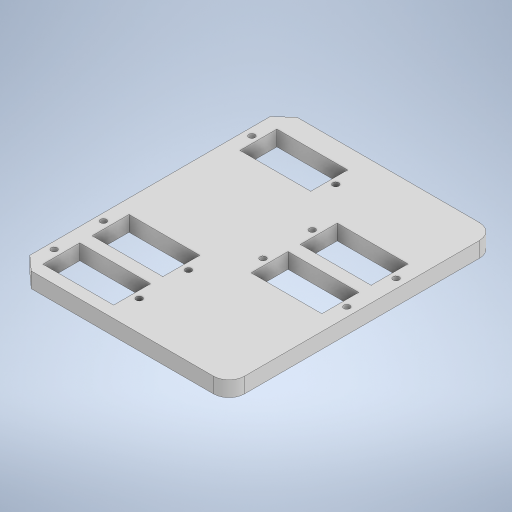
# Autodesk Inventor part: Robotic Hand Tray
Saved by Autodesk Inventor 2023 (Build 270158000, 158)
## iProperties
Created: 2023-03-10
Part Number: Robotic Hand Tray
Material: Generic
Document SubType Name: Modeling
Designer: 1senadi
Density: 1 g/cm^3
Appearance: Default
Author: 1senadi
Autodesk Inventor part; units mm, degrees
ref_plane "YZ Plane" through (0, 0, 0) normal (1, 0, 0) x (0, 1, 0)
ref_plane "XZ Plane" through (0, 0, 0) normal (0, 1, 0) x (-1, 0, 0)
ref_plane "Work Plane2" through (0, 5.93, 0) normal (0, 1, 0) x (1, 0, 0)
sketch "Sketch7" plane through (0, 5.93, 0) normal (0, 1, 0) x (1, 0, 0)
  line L0 (-68.89, 72.25) -> (-68.89, 75.38) projected
  line L1 (-70.59, 75.38) -> (-68.89, 75.38) projected
  line L2 (-70.59, 83.0068) -> (-70.59, 75.38) projected
  line L3 (-64.9127, 88.12) -> (-70.59, 83.0068) projected
  line L4 (-5, 88.12) -> (-64.9127, 88.12) projected
  arc A0 (1.7, 81.42) -> (-5, 88.12) centre (-5, 81.42) ccw projected
  line L5 (1.7, 5) -> (1.7, 81.42) projected
  arc A1 (-5, -1.7) -> (1.7, 5) centre (-5, 5) ccw projected
  line L6 (-64.9127, -1.7) -> (-5, -1.7) projected
  line L7 (-70.59, 3.4132) -> (-64.9127, -1.7) projected
  line L8 (-70.59, 14.5) -> (-70.59, 3.4132) projected
  line L9 (-68.89, 14.5) -> (-70.59, 14.5) projected
  line L10 (-68.89, 14.5) -> (-68.89, 17.63) projected
  line L11 (-70.59, 17.63) -> (-68.89, 17.63) projected
  line L12 (-70.59, 47.6) -> (-70.59, 17.63) projected
  line L13 (-68.89, 47.6) -> (-70.59, 47.6) projected
  line L14 (-68.89, 47.6) -> (-68.89, 50.73) projected
  line L15 (-70.59, 50.73) -> (-68.89, 50.73) projected
  line L16 (-70.59, 72.25) -> (-70.59, 50.73) projected
  line L17 (-68.89, 72.25) -> (-70.59, 72.25) projected
  line L18 (5.3534, 92.34) -> (10.14, 87.0271) projected
  line L19 (-69.6869, 92.34) -> (5.3534, 92.34) projected
  line L20 (-73.78, 86.0365) -> (-69.6869, 92.34) projected
  line L21 (-73.78, 75.38) -> (-73.78, 86.0365) projected
  line L22 (-73.78, 75.38) -> (-73.78, 72.25) projected
  line L23 (-73.78, 50.73) -> (-73.78, 72.25) projected
  line L24 (-73.78, 50.73) -> (-73.78, 47.6) projected
  line L25 (-73.78, 17.63) -> (-73.78, 47.6) projected
  line L26 (-73.78, 17.63) -> (-73.78, 14.5) projected
  line L27 (-73.78, -2.6865) -> (-73.78, 14.5) projected
  line L28 (-69.6869, -8.99) -> (-73.78, -2.6865) projected
  line L29 (4.8271, -8.99) -> (-69.6869, -8.99) projected
  line L30 (10.14, -4.2034) -> (4.8271, -8.99) projected
  line L31 (10.14, 87.0271) -> (10.14, -4.2034) projected
  line L32 (-5, 0) -> (-64.26, 0) projected
  line L33 (-68.89, 4.17) -> (-64.26, 0) projected
  line L34 (-68.89, 4.17) -> (-68.89, 14.5) projected
  line L35 (-68.89, 17.63) -> (-68.89, 47.6) projected
  line L36 (-68.89, 50.73) -> (-68.89, 72.25) projected
  line L37 (-68.89, 75.38) -> (-68.89, 82.25) projected
  line L38 (-64.26, 86.42) -> (-68.89, 82.25) projected
  line L39 (-64.26, 86.42) -> (-5, 86.42) projected
  arc A2 (0, 81.42) -> (-5, 86.42) centre (-5, 81.42) ccw projected
  line L40 (0, 81.42) -> (0, 5) projected
  arc A3 (-5, 0) -> (0, 5) centre (-5, 5) ccw projected
  line L41 (-68.89, 14.5) -> (-70.59, 14.5) projected
  line L42 (-68.89, 14.5) -> (-68.89, 75.38)
  point P0 (0, 0)
  constraints: 2 end point, 1 collinear
extrude "Extrusion6" add sketch "Sketch7" along normal blind 5 contours L0 L37 L38 L39 A2 L40 A3 L32 L33 L34 L10 L35 L14 L36
sketch "Sketch8" plane through (0, 10.93, 0) normal (0, 1, 0) x (1, 0, 0)
  line L0 (-64.26, 0) -> (-64.26, 16.2)
  line L1 (-64.26, 16.2) -> (-64.26, 17.765)
  line L2 (-64.26, 17.765) -> (-41.26, 17.765)
  line L3 (-64.26, 17.765) -> (-64.26, 15.765)
  line L4 (-64.26, 15.765) -> (-41.26, 15.765)
  line L5 (-41.26, 15.765) -> (-41.26, 3.765)
  line L6 (-41.26, 3.765) -> (-64.26, 3.765)
  line L7 (-64.26, 3.765) -> (-64.26, 15.765)
  line L8 (-64.26, 9.765) -> (-66.573, 9.765)
  circle A0 centre (-66.573, 9.765) radius 1
  line L9 (-41.26, 9.765) -> (-38.947, 9.765)
  circle A1 centre (-38.947, 9.765) radius 1
  line L10 (-64.26, 17.765) -> (-64.26, 19.765)
  line L11 (-64.26, 19.765) -> (-41.26, 19.765)
  line L12 (-41.26, 19.765) -> (-41.26, 31.765)
  line L13 (-41.26, 31.765) -> (-64.26, 31.765)
  line L14 (-64.26, 31.765) -> (-64.26, 19.765)
  line L15 (-64.26, 25.765) -> (-66.573, 25.765)
  circle A2 centre (-66.573, 25.765) radius 1
  line L16 (-41.26, 25.765) -> (-38.947, 25.765)
  circle A3 centre (-38.947, 25.765) radius 1
  point P0 (0, 0)
  dimension "d56" = 16.2
  dimension "d57" = 1.565
  dimension "d58" = 23
  dimension "d59" = 90
  dimension "d60" = 2
  dimension "d61" = 23
  dimension "d62" = 12
  dimension "d63" = 2.313
  dimension "d64" = 2
  dimension "d65" = 2.313
  dimension "d66" = 2
  dimension "d67" = 2
  dimension "d68" = 23
  dimension "d69" = 12
  dimension "d70" = 2.313
  dimension "d71" = 2
  dimension "d73" = 2
  constraints: 34 end point, 6 horizontal, 4 centre point, 4 coincident, 4 midpoint, 4 parallel, 3 perpendicular, 3 vertical, 1 point on line
  measures "d56" distance of L0.start L0.end
  measures "d57" distance of L0.end L1.end
  measures "d58" distance of L1.end L2.end
  measures "d59" angle of L1 L2
  measures "d60" distance of L1.end L3.end
  measures "d61" distance of L5.end L6.end
  measures "d62" distance of L4.end L5.end
  measures "d63" distance of L8.start L8.end
  measures "d64" diameter of A0
  measures "d65" distance of L9.start L9.end
  measures "d66" diameter of A1
  measures "d67" distance of L1.end L10.end
  measures "d68" distance of L13.end L12.end
  measures "d69" distance of L12.end L11.end
  measures "d70" distance of L15.start L15.end
  measures "d71" diameter of A2
  measures "d73" diameter of A3
extrude "Extrusion7" cut sketch "Sketch8" against normal up to surface (5 mm away)
sketch "Sketch9" plane through (0, 10.93, 0) normal (0, 1, 0) x (1, 0, 0)
  line L0 (-5, 86.42) -> (-64.26, 86.42) projected
  line L1 (-64.26, 86.42) -> (-64.26, 75.38)
  line L2 (-64.26, 75.38) -> (-64.26, 73.815)
  line L3 (-64.26, 73.815) -> (-64.26, 79.815)
  line L4 (-64.26, 79.815) -> (-41.26, 79.815)
  line L5 (-64.26, 73.815) -> (-66.39, 73.815)
  circle A0 centre (-66.39, 73.815) radius 1
  line L6 (-41.26, 79.815) -> (-41.26, 67.815)
  line L7 (-41.26, 67.815) -> (-64.26, 67.815)
  line L8 (-64.26, 67.815) -> (-64.26, 73.815)
  line L9 (-41.26, 73.815) -> (-39.13, 73.815)
  circle A1 centre (-39.13, 73.815) radius 1
  point P0 (0, 0)
  dimension "d76" = 11.04
  dimension "d77" = 1.565
  dimension "d79" = 6
  dimension "d80" = 23
  dimension "d82" = 2.13
  dimension "d85" = 2
  dimension "d88" = 12
  dimension "d89" = 23
  dimension "d90" = 2.13
  dimension "d91" = 2
  constraints: 18 end point, 3 vertical, 2 centre point, 2 coincident, 2 horizontal, 2 perpendicular, 1 midpoint, 1 point on line
  measures "d76" distance of L0.end L1.end
  measures "d77" distance of L1.end L2.end
  measures "d79" distance of L2.end L3.end
  measures "d80" distance of L3.end L4.end
  measures "d82" distance of L2.end L5.end
  measures "d85" diameter of A0
  measures "d88" distance of L4.end L6.end
  measures "d89" distance of L6.end L7.end
  measures "d90" distance of L9.start L9.end
  measures "d91" diameter of A1
extrude "Extrusion8" cut sketch "Sketch9" against normal up to surface (5 mm away)
sketch "Sketch10" plane through (0, 10.93, 0) normal (0, 1, 0) x (1, 0, 0)
  arc A0 (0, 81.42) -> (-5, 86.42) centre (-5, 81.42) ccw projected
  line L0 (0, 81.42) -> (0, 49.165)
  line L1 (0, 49.165) -> (-5, 49.165)
  line L2 (-5, 49.165) -> (-5, 51.165)
  line L3 (-5, 49.165) -> (-5, 47.165)
  line L4 (-5, 51.165) -> (-28, 51.165)
  line L5 (-28, 51.165) -> (-28, 63.165)
  line L6 (-28, 63.165) -> (-5, 63.165)
  line L7 (-5, 63.165) -> (-5, 51.165)
  line L8 (-5, 47.165) -> (-28, 47.165)
  line L9 (-28, 47.165) -> (-28, 35.165)
  line L10 (-28, 35.165) -> (-5, 35.165)
  line L11 (-5, 35.165) -> (-5, 47.165)
  line L12 (-28, 41.165) -> (-30.13, 41.165)
  line L13 (-5, 41.165) -> (-2.87, 41.165)
  circle A1 centre (-30.13, 41.165) radius 1
  circle A2 centre (-2.87, 41.165) radius 1
  line L14 (-28, 57.165) -> (-30.13, 57.165)
  line L15 (-5, 57.165) -> (-2.87, 57.165)
  circle A3 centre (-30.13, 57.165) radius 1
  circle A4 centre (-2.87, 57.165) radius 1
  point P0 (0, 0)
  dimension "d92" = 32.255
  dimension "d93" = 5
  dimension "d94" = 2
  dimension "d95" = 2
  dimension "d96" = 23
  dimension "d97" = 12
  dimension "d98" = 23
  dimension "d99" = 12
  dimension "d100" = 2.13
  dimension "d101" = 2.13
  dimension "d102" = 2
  dimension "d103" = 2
  dimension "d104" = 2.13
  dimension "d105" = 2.13
  dimension "d106" = 2
  dimension "d107" = 2
  constraints: 32 end point, 6 horizontal, 4 centre point, 4 coincident, 4 midpoint, 4 parallel, 4 perpendicular, 2 vertical, 1 tangent
  measures "d92" distance of L0.start L0.end
  measures "d93" distance of L0.end L1.end
  measures "d94" distance of L1.end L2.end
  measures "d95" distance of L1.end L3.end
  measures "d96" distance of L5.end L6.end
  measures "d97" distance of L4.end L5.end
  measures "d98" distance of L10.end L9.end
  measures "d99" distance of L9.end L8.end
  measures "d100" distance of L12.start L12.end
  measures "d101" distance of L13.start L13.end
  measures "d102" diameter of A1
  measures "d103" diameter of A2
  measures "d104" distance of L14.start L14.end
  measures "d105" distance of L15.start L15.end
  measures "d106" diameter of A3
  measures "d107" diameter of A4
extrude "Extrusion9" cut sketch "Sketch10" against normal up to surface (5 mm away)
body "Solid1"
